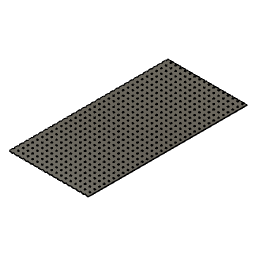
plate v1 (Autodesk Fusion 360 design; units mm, degrees)
Autodesk Fusion 360 part; units mm, degrees
sketch "Sketch1" plane through (0, 0, 0) normal (0, 0, 1) x (1, 0, 0)
  line L0 (0, 0) -> (250, 0)
  line L1 (250, 0) -> (250, 500)
  line L2 (250, 500) -> (0, 500)
  line L3 (0, 500) -> (0, 0)
  dimension "d1" = 500
  dimension "d2" = 250
  constraint horizontal L0
  constraint vertical L1
  constraint horizontal L2
  constraint vertical L3
  constraint coincident L0.start L3.end
  measures "d1" distance of L0.start L2.end
  measures "d2" distance of L0.start L0.end
extrude "Extrude1" add sketch "Sketch1" along normal blind 1.5
sketch "Sketch2" plane through (0, 0, 1.5) normal (0, 0, 1) x (-1, 0, 0)
  line L0 (0, -500) -> (0, 0)
  line L1 (0, 0) -> (-250, 0)
  line L2 (-250, 0) -> (-250, -500)
  line L3 (-250, -500) -> (0, -500)
  circle A0 centre (0, 0) radius 2.25
  dimension "d5" = 4.5
  constraint coincident L0.end L1.start
  measures "d5" diameter of A0
extrude "Extrude2" cut sketch "Sketch2" against normal up to surface (1.5 mm away) contours L0 L1 A0 | L0 L1 A0
pattern_linear "R-Pattern1" count 34 spacing 15 along (0, 1, 0) count 17 spacing 15 along (1, 0, 0) of "Extrude2"
